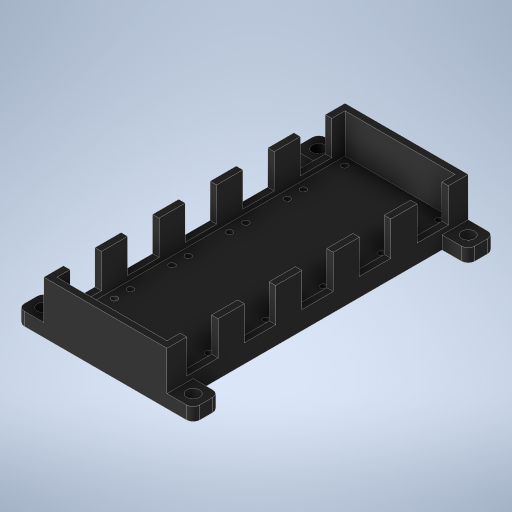
# Autodesk Inventor part: RelayCaseBottom
Saved by Autodesk Inventor 2024 (Build 280153000, 153)
## iProperties
Created: 2023-08-11
Part Number: RelayCaseBottom
Material: Rubber, Silicone
Document SubType Name: Modeling
Designer: 18179
Density: 1.25 g/cm^3
Appearance: Rubber - Black
Autodesk Inventor part; units mm, degrees
ref_plane "YZ Plane" through (0, 0, 0) normal (1, 0, 0) x (0, 1, 0)
ref_plane "XZ Plane" through (0, 0, 0) normal (0, 1, 0) x (-1, 0, 0)
ref_plane "XY Plane" through (0, 0, 0) normal (0, 0, 1) x (1, 0, 0)
sketch "0" plane through (0, 0, 0) normal (0, 0, 1) x (1, 0, 0)
  line L0 (-55.1011, 34.3581) -> (-55.1011, 26.7381)
  line L1 (-55.1011, 26.7381) -> (-57.6411, 26.7381)
  line L2 (-57.6411, 26.7381) -> (-57.6411, 34.3581)
  line L3 (-57.6411, 34.3581) -> (-55.1011, 34.3581)
  line L4 (-53.2169, 46.974) -> (-78.6169, 46.974)
  line L5 (-78.6169, 46.974) -> (-78.6169, -3.826)
  line L6 (-78.6169, -3.826) -> (-53.2169, -3.826)
  line L7 (-53.2169, -3.826) -> (-53.2169, 46.974)
  line L8 (-73.5115, 6.588) -> (-73.5115, 24.368)
  line L9 (-73.5115, 24.368) -> (-58.3223, 24.368)
  line L10 (-58.3223, 24.368) -> (-58.3223, 6.588)
  line L11 (-58.3223, 6.588) -> (-58.2969, 6.588)
  line L12 (-58.2969, 6.588) -> (-58.2969, -1.159)
  line L13 (-58.2969, -1.159) -> (-73.5369, -1.159)
  line L14 (-73.5369, -1.159) -> (-73.5369, 6.588)
  line L15 (-73.5369, 6.588) -> (-73.5115, 6.588)
  line L16 (-73.5369, 37.449) -> (-73.5369, 45.196)
  line L17 (-73.5369, 45.196) -> (-58.2969, 45.196)
  line L18 (-58.2969, 45.196) -> (-58.2969, 37.449)
  line L19 (-58.2969, 37.449) -> (-73.5369, 37.449)
  circle A0 centre (-75.9499, -1.2407) radius 1.524
  circle A1 centre (-55.8839, -1.2407) radius 1.524
  circle A2 centre (-75.9499, 44.3888) radius 1.524
  circle A3 centre (-55.8839, 44.3888) radius 1.524
  line L20 (-83.0411, 34.3581) -> (-83.0411, 26.7381)
  line L21 (-83.0411, 26.7381) -> (-85.5811, 26.7381)
  line L22 (-85.5811, 26.7381) -> (-85.5811, 34.3581)
  line L23 (-85.5811, 34.3581) -> (-83.0411, 34.3581)
  line L24 (-81.1569, 46.974) -> (-106.5569, 46.974)
  line L25 (-106.5569, 46.974) -> (-106.5569, -3.826)
  line L26 (-106.5569, -3.826) -> (-81.1569, -3.826)
  line L27 (-81.1569, -3.826) -> (-81.1569, 46.974)
  line L28 (-101.4515, 6.588) -> (-101.4515, 24.368)
  line L29 (-101.4515, 24.368) -> (-86.2623, 24.368)
  line L30 (-86.2623, 24.368) -> (-86.2623, 6.588)
  line L31 (-86.2623, 6.588) -> (-86.2369, 6.588)
  line L32 (-86.2369, 6.588) -> (-86.2369, -1.159)
  line L33 (-86.2369, -1.159) -> (-101.4769, -1.159)
  line L34 (-101.4769, -1.159) -> (-101.4769, 6.588)
  line L35 (-101.4769, 6.588) -> (-101.4515, 6.588)
  line L36 (-101.4769, 37.449) -> (-101.4769, 45.196)
  line L37 (-101.4769, 45.196) -> (-86.2369, 45.196)
  line L38 (-86.2369, 45.196) -> (-86.2369, 37.449)
  line L39 (-86.2369, 37.449) -> (-101.4769, 37.449)
  circle A4 centre (-103.8899, -1.2407) radius 1.524
  circle A5 centre (-83.8239, -1.2407) radius 1.524
  circle A6 centre (-103.8899, 44.3888) radius 1.524
  circle A7 centre (-83.8239, 44.3888) radius 1.524
  line L40 (-110.9811, 34.3581) -> (-110.9811, 26.7381)
  line L41 (-110.9811, 26.7381) -> (-113.5211, 26.7381)
  line L42 (-113.5211, 26.7381) -> (-113.5211, 34.3581)
  line L43 (-113.5211, 34.3581) -> (-110.9811, 34.3581)
  line L44 (-109.0969, 46.974) -> (-134.4969, 46.974)
  line L45 (-134.4969, 46.974) -> (-134.4969, -3.826)
  line L46 (-134.4969, -3.826) -> (-109.0969, -3.826)
  line L47 (-109.0969, -3.826) -> (-109.0969, 46.974)
  line L48 (-129.3915, 6.588) -> (-129.3915, 24.368)
  line L49 (-129.3915, 24.368) -> (-114.2023, 24.368)
  line L50 (-114.2023, 24.368) -> (-114.2023, 6.588)
  line L51 (-114.2023, 6.588) -> (-114.1769, 6.588)
  line L52 (-114.1769, 6.588) -> (-114.1769, -1.159)
  line L53 (-114.1769, -1.159) -> (-129.4169, -1.159)
  line L54 (-129.4169, -1.159) -> (-129.4169, 6.588)
  line L55 (-129.4169, 6.588) -> (-129.3915, 6.588)
  line L56 (-129.4169, 37.449) -> (-129.4169, 45.196)
  line L57 (-129.4169, 45.196) -> (-114.1769, 45.196)
  line L58 (-114.1769, 45.196) -> (-114.1769, 37.449)
  line L59 (-114.1769, 37.449) -> (-129.4169, 37.449)
  circle A8 centre (-131.8299, -1.2407) radius 1.524
  circle A9 centre (-111.7639, -1.2407) radius 1.524
  circle A10 centre (-131.8299, 44.3888) radius 1.524
  circle A11 centre (-111.7639, 44.3888) radius 1.524
  line L60 (-138.9211, 34.3581) -> (-138.9211, 26.7381)
  line L61 (-138.9211, 26.7381) -> (-141.4611, 26.7381)
  line L62 (-141.4611, 26.7381) -> (-141.4611, 34.3581)
  line L63 (-141.4611, 34.3581) -> (-138.9211, 34.3581)
  line L64 (-137.0369, 46.974) -> (-162.4369, 46.974)
  line L65 (-162.4369, 46.974) -> (-162.4369, -3.826)
  line L66 (-162.4369, -3.826) -> (-137.0369, -3.826)
  line L67 (-137.0369, -3.826) -> (-137.0369, 46.974)
  line L68 (-157.3315, 6.588) -> (-157.3315, 24.368)
  line L69 (-157.3315, 24.368) -> (-142.1423, 24.368)
  line L70 (-142.1423, 24.368) -> (-142.1423, 6.588)
  line L71 (-142.1423, 6.588) -> (-142.1169, 6.588)
  line L72 (-142.1169, 6.588) -> (-142.1169, -1.159)
  line L73 (-142.1169, -1.159) -> (-157.3569, -1.159)
  line L74 (-157.3569, -1.159) -> (-157.3569, 6.588)
  line L75 (-157.3569, 6.588) -> (-157.3315, 6.588)
  line L76 (-157.3569, 37.449) -> (-157.3569, 45.196)
  line L77 (-157.3569, 45.196) -> (-142.1169, 45.196)
  line L78 (-142.1169, 45.196) -> (-142.1169, 37.449)
  line L79 (-142.1169, 37.449) -> (-157.3569, 37.449)
  circle A12 centre (-159.7699, -1.2407) radius 1.524
  circle A13 centre (-139.7039, -1.2407) radius 1.524
  circle A14 centre (-159.7699, 44.3888) radius 1.524
  circle A15 centre (-139.7039, 44.3888) radius 1.524
  line L80 (-166.8611, 34.3581) -> (-166.8611, 26.7381)
  line L81 (-166.8611, 26.7381) -> (-169.4011, 26.7381)
  line L82 (-169.4011, 26.7381) -> (-169.4011, 34.3581)
  line L83 (-169.4011, 34.3581) -> (-166.8611, 34.3581)
  line L84 (-164.9769, 46.974) -> (-190.3769, 46.974)
  line L85 (-190.3769, 46.974) -> (-190.3769, -3.826)
  line L86 (-190.3769, -3.826) -> (-164.9769, -3.826)
  line L87 (-164.9769, -3.826) -> (-164.9769, 46.974)
  line L88 (-185.2715, 6.588) -> (-185.2715, 24.368)
  line L89 (-185.2715, 24.368) -> (-170.0823, 24.368)
  line L90 (-170.0823, 24.368) -> (-170.0823, 6.588)
  line L91 (-170.0823, 6.588) -> (-170.0569, 6.588)
  line L92 (-170.0569, 6.588) -> (-170.0569, -1.159)
  line L93 (-170.0569, -1.159) -> (-185.2969, -1.159)
  line L94 (-185.2969, -1.159) -> (-185.2969, 6.588)
  line L95 (-185.2969, 6.588) -> (-185.2715, 6.588)
  line L96 (-185.2969, 37.449) -> (-185.2969, 45.196)
  line L97 (-185.2969, 45.196) -> (-170.0569, 45.196)
  line L98 (-170.0569, 45.196) -> (-170.0569, 37.449)
  line L99 (-170.0569, 37.449) -> (-185.2969, 37.449)
  circle A16 centre (-187.7099, -1.2407) radius 1.524
  circle A17 centre (-167.6439, -1.2407) radius 1.524
  circle A18 centre (-187.7099, 44.3888) radius 1.524
  circle A19 centre (-167.6439, 44.3888) radius 1.524
  line L100 (-53.2169, -3.826) -> (-190.3769, -3.826)
  line L101 (-190.3769, -3.826) -> (-190.3769, 46.974)
  line L102 (-190.3769, 46.974) -> (-53.2169, 46.974)
  line L103 (-53.2169, 46.974) -> (-53.2169, -3.826)
  line L104 (-190.3769, 47.736) -> (-52.4549, 47.736)
  line L105 (-52.4549, 47.736) -> (-52.4549, -3.826)
  line L106 (-53.2169, -4.588) -> (-191.1389, -4.588)
  line L107 (-191.1389, -4.588) -> (-191.1389, 46.974)
  line L108 (-191.1389, -4.588) -> (-52.4549, -4.588)
  line L109 (-52.4549, -4.588) -> (-52.4549, 47.736)
  line L110 (-52.4549, 47.736) -> (-191.1389, 47.736)
  line L111 (-191.1389, 47.736) -> (-191.1389, -4.588)
  point P0 (-73.5369, 45.196)
  point P1 (-53.2169, -4.588)
  point P2 (-52.4549, -3.826)
  point P3 (-101.4769, 37.449)
  point P4 (-101.4769, -1.159)
  point P5 (-101.4769, 6.588)
  point P6 (-101.4515, 6.588)
  point P7 (-157.3569, 6.588)
  point P8 (-142.1169, 6.588)
  point P9 (-73.5115, 6.588)
  point P10 (-58.2969, -1.159)
  dimension "d0" = 25.4
  dimension "d1" = 50.8
  dimension "d2" = 3.048
  dimension "d3" = 1.8843
  dimension "d4" = 4.4243
  dimension "d5" = 5.08
  dimension "d6" = 5.08
  dimension "d7" = 5.1054
  dimension "d8" = 20.2946
  dimension "d9" = 20.32
  dimension "d10" = 20.32
  dimension "d11" = 7.62
  dimension "d12" = 12.6159
  dimension "d13" = 10.8379
  dimension "d14" = 3.0909
  dimension "d15" = 9.9901
  dimension "d16" = 35.5171
  dimension "d17" = 27.7701
  dimension "d18" = 20.1501
  dimension "d19" = 12.6159
  dimension "d20" = 0
  dimension "d21" = 38.1841
  dimension "d22" = 0
  dimension "d23" = 0
  dimension "d24" = 1.8843
  dimension "d25" = 7.62
  dimension "d26" = 1.8843
  dimension "d27" = 2.667
  dimension "d28" = 10.0307
  dimension "d29" = 2.667
  dimension "d30" = 35.5988
  dimension "d31" = 0
  dimension "d32" = 4.4243
  dimension "d33" = 7.62
  dimension "d34" = 4.4243
  dimension "d35" = 10.8379
  dimension "d36" = 5.08
  dimension "d37" = 3.0909
  dimension "d38" = 5.08
  dimension "d39" = 5.08
  dimension "d40" = 27.7701
  dimension "d41" = 5.08
  dimension "d42" = 35.5171
  dimension "d43" = 9.9901
  dimension "d44" = 5.1054
  dimension "d45" = 5.1054
  dimension "d46" = 27.7701
  dimension "d47" = 9.9901
  dimension "d48" = 20.2946
  dimension "d49" = 27.7701
  dimension "d50" = 20.2946
  dimension "d51" = 10.8379
  dimension "d52" = 20.32
  dimension "d53" = 3.0909
  dimension "d54" = 20.32
  dimension "d55" = 20.32
  dimension "d56" = 27.7701
  dimension "d57" = 20.32
  dimension "d58" = 35.5171
  dimension "d59" = 22.733
  dimension "d60" = 10.0307
  dimension "d61" = 22.733
  dimension "d62" = 35.5988
  dimension "d63" = 25.4
  constraints: 224 end point, 44 parallel, 38 perpendicular, 20 centre point, 15 equal radius, 14 collinear, 2 horizontal, 2 other
  measures "d0" distance between parallel lines of L7 L5
  measures "d1" distance between parallel lines of L6 L4
  measures "d2" diameter of A3
  measures "d3" distance between parallel lines of L0 L7
  measures "d4" distance between parallel lines of L2 L7
  measures "d5" distance between parallel lines of L7 L18
  measures "d6" distance between parallel lines of L12 L7
  measures "d7" distance between parallel lines of L7 L10
  measures "d8" distance between parallel lines of L7 L8
  measures "d9" distance between parallel lines of L7 L16
  measures "d10" distance between parallel lines of L14 L7
  measures "d11" distance between parallel lines of L1 L3
  measures "d12" distance between parallel lines of L3 L4
  measures "d13" distance between parallel lines of L3 L17
  measures "d14" distance between parallel lines of L3 L19
  measures "d15" distance between parallel lines of L3 L9
  measures "d16" distance between parallel lines of L13 L3
  measures "d17" distance between parallel lines of L3 L15
  measures "d18" distance between parallel lines of L11 L1
  measures "d19" distance from line of L7.end L3
  measures "d20" distance from line of L4.start L7
  measures "d21" distance from line of L7.start L3
  measures "d22" distance from line of L6.end L7
  measures "d23" distance from line of L0.start L3
  measures "d24" distance from line of L3.end L7
  measures "d25" distance from line of L0.end L3
  measures "d26" distance from line of L1.start L7
  measures "d27" distance from line of A3.centre L7
  measures "d28" distance from line of A3.centre L3
  measures "d29" distance from line of A1.centre L7
  measures "d30" distance from line of A1.centre L3
  measures "d31" distance from line of L2.end L3
  measures "d32" distance from line of L3.start L7
  measures "d33" distance from line of L2.start L3
  measures "d34" distance from line of L1.end L7
  measures "d35" distance from line of L18.start L3
  measures "d36" distance from line of L17.end L7
  measures "d37" distance from line of L18.end L3
  measures "d38" distance from line of L19.start L7
  measures "d39" distance from line of L11.end L7
  measures "d40" distance from line of L12.start L3
  measures "d41" distance from line of L13.start L7
  measures "d42" distance from line of L12.end L3
  measures "d43" distance from line of L10.start L3
  measures "d44" distance from line of L9.end L7
  measures "d45" distance from line of L11.start L7
  measures "d46" distance from line of L10.end L3
  measures "d47" distance from line of L8.end L3
  measures "d48" distance from line of L9.start L7
  measures "d49" distance from line of L8.start L3
  measures "d50" distance from line of L15.end L7
  measures "d51" distance from line of L16.end L3
  measures "d52" distance from line of L17.start L7
  measures "d53" distance from line of L16.start L3
  measures "d54" distance from line of L19.end L7
  measures "d55" distance from line of L15.start L7
  measures "d56" distance from line of L14.end L3
  measures "d57" distance from line of L13.end L7
  measures "d58" distance from line of L14.start L3
  measures "d59" distance from line of A2.centre L7
  measures "d60" distance from line of A2.centre L3
  measures "d61" distance from line of A0.centre L7
  measures "d62" distance from line of A0.centre L3
  measures "d63" distance from line of L4.end L7
extrude "Extrusion1" add sketch "0" along normal blind 3.175 contours L0 L1 L2 L3 | L7 L6 L5 L4 | L5 L100 L27 L102 | L27 L26 L25 L24 | L25 L100 L47 L102 | L47 L46 L45 L44 | L45 L100 L67 L102 | L67 L66 L65 L64 | L65 L100 L87 L102 | L87 L86 L85 L84 | L20 L21 L22 L23 | L40 L41 L42 L43 | L60 L61 L62 L63 | L80 L81 L82 L83 | L104 L105 L109 L108 L106 L107 L111 L110
sketch "Sketch10" plane through (0, 0, 3.175) normal (0, 0, 1) x (1, 0, 0)
  line L0 (-191.1389, 47.736) -> (-191.1389, -4.588) projected
  line L1 (-191.1389, -4.588) -> (-52.4549, -4.588) projected
  line L2 (-52.4549, -4.588) -> (-52.4549, 47.736) projected
  line L3 (-52.4549, 47.736) -> (-191.1389, 47.736) projected
  line L4 (-101.4769, -1.159) -> (-101.4769, 6.588) projected
  line L5 (-101.4769, 6.588) -> (-101.4515, 6.588) projected
  line L6 (-101.4515, 6.588) -> (-101.4515, 24.368) projected
  line L7 (-101.4515, 24.368) -> (-86.2623, 24.368) projected
  line L8 (-86.2623, 24.368) -> (-86.2623, 6.588) projected
  line L9 (-86.2623, 6.588) -> (-86.2369, 6.588) projected
  line L10 (-86.2369, 6.588) -> (-86.2369, -1.159) projected
  line L11 (-86.2369, -1.159) -> (-101.4769, -1.159) projected
  line L12 (-86.2369, 37.449) -> (-101.4769, 37.449) projected
  line L13 (-101.4769, 37.449) -> (-101.4769, 45.196) projected
  line L14 (-101.4769, 45.196) -> (-86.2369, 45.196) projected
  line L15 (-86.2369, 45.196) -> (-86.2369, 37.449) projected
  circle A0 centre (-103.8899, 44.3888) radius 1.524 projected
  circle A1 centre (-83.8239, 44.3888) radius 1.524 projected
  circle A2 centre (-103.8899, -1.2407) radius 1.524 projected
  circle A3 centre (-83.8239, -1.2407) radius 1.524 projected
  line L16 (-157.3569, -1.159) -> (-157.3569, 6.588) projected
  line L17 (-157.3569, 6.588) -> (-157.3315, 6.588) projected
  line L18 (-157.3315, 6.588) -> (-157.3315, 24.368) projected
  line L19 (-157.3315, 24.368) -> (-142.1423, 24.368) projected
  line L20 (-142.1423, 24.368) -> (-142.1423, 6.588) projected
  line L21 (-142.1423, 6.588) -> (-142.1169, 6.588) projected
  line L22 (-142.1169, 6.588) -> (-142.1169, -1.159) projected
  line L23 (-142.1169, -1.159) -> (-157.3569, -1.159) projected
  line L24 (-142.1169, 37.449) -> (-157.3569, 37.449) projected
  line L25 (-157.3569, 37.449) -> (-157.3569, 45.196) projected
  line L26 (-157.3569, 45.196) -> (-142.1169, 45.196) projected
  line L27 (-142.1169, 45.196) -> (-142.1169, 37.449) projected
  circle A4 centre (-159.7699, 44.3888) radius 1.524 projected
  circle A5 centre (-139.7039, 44.3888) radius 1.524 projected
  circle A6 centre (-159.7699, -1.2407) radius 1.524 projected
  circle A7 centre (-139.7039, -1.2407) radius 1.524 projected
  line L28 (-185.2969, -1.159) -> (-185.2969, 6.588) projected
  line L29 (-185.2969, 6.588) -> (-185.2715, 6.588) projected
  line L30 (-185.2715, 6.588) -> (-185.2715, 24.368) projected
  line L31 (-185.2715, 24.368) -> (-170.0823, 24.368) projected
  line L32 (-170.0823, 24.368) -> (-170.0823, 6.588) projected
  line L33 (-170.0823, 6.588) -> (-170.0569, 6.588) projected
  line L34 (-170.0569, 6.588) -> (-170.0569, -1.159) projected
  line L35 (-170.0569, -1.159) -> (-185.2969, -1.159) projected
  line L36 (-170.0569, 37.449) -> (-185.2969, 37.449) projected
  line L37 (-185.2969, 37.449) -> (-185.2969, 45.196) projected
  line L38 (-185.2969, 45.196) -> (-170.0569, 45.196) projected
  line L39 (-170.0569, 45.196) -> (-170.0569, 37.449) projected
  circle A8 centre (-187.7099, 44.3888) radius 1.524 projected
  circle A9 centre (-167.6439, 44.3888) radius 1.524 projected
  circle A10 centre (-187.7099, -1.2407) radius 1.524 projected
  circle A11 centre (-167.6439, -1.2407) radius 1.524 projected
  circle A12 centre (-111.7639, -1.2407) radius 1.524 projected
  circle A13 centre (-131.8299, -1.2407) radius 1.524 projected
  circle A14 centre (-111.7639, 44.3888) radius 1.524 projected
  circle A15 centre (-131.8299, 44.3888) radius 1.524 projected
  line L40 (-114.1769, 37.449) -> (-129.4169, 37.449) projected
  line L41 (-129.4169, 37.449) -> (-129.4169, 45.196) projected
  line L42 (-129.4169, 45.196) -> (-114.1769, 45.196) projected
  line L43 (-114.1769, 45.196) -> (-114.1769, 37.449) projected
  line L44 (-129.4169, -1.159) -> (-129.4169, 6.588) projected
  line L45 (-129.4169, 6.588) -> (-129.3915, 6.588) projected
  line L46 (-129.3915, 6.588) -> (-129.3915, 24.368) projected
  line L47 (-129.3915, 24.368) -> (-114.2023, 24.368) projected
  line L48 (-114.2023, 24.368) -> (-114.2023, 6.588) projected
  line L49 (-114.2023, 6.588) -> (-114.1769, 6.588) projected
  line L50 (-114.1769, 6.588) -> (-114.1769, -1.159) projected
  line L51 (-114.1769, -1.159) -> (-129.4169, -1.159) projected
  line L52 (-73.5115, 6.588) -> (-73.5115, 24.368) projected
  line L53 (-73.5115, 24.368) -> (-58.3223, 24.368) projected
  line L54 (-58.3223, 24.368) -> (-58.3223, 6.588) projected
  line L55 (-58.3223, 6.588) -> (-58.2969, 6.588) projected
  line L56 (-58.2969, 6.588) -> (-58.2969, -1.159) projected
  line L57 (-58.2969, -1.159) -> (-73.5369, -1.159) projected
  line L58 (-73.5369, -1.159) -> (-73.5369, 6.588) projected
  line L59 (-73.5369, 6.588) -> (-73.5115, 6.588) projected
  line L60 (-73.5369, 37.449) -> (-73.5369, 45.196) projected
  line L61 (-73.5369, 45.196) -> (-58.2969, 45.196) projected
  line L62 (-58.2969, 45.196) -> (-58.2969, 37.449) projected
  line L63 (-58.2969, 37.449) -> (-73.5369, 37.449) projected
  circle A16 centre (-55.8839, 44.3888) radius 1.524 projected
  circle A17 centre (-75.9499, 44.3888) radius 1.524 projected
  circle A18 centre (-55.8839, -1.2407) radius 1.524 projected
  circle A19 centre (-75.9499, -1.2407) radius 1.524 projected
  line L64 (-191.6865, 48.2837) -> (-191.6865, -5.1356)
  line L65 (-191.6865, -5.1356) -> (-51.9072, -5.1356)
  line L66 (-51.9072, -5.1356) -> (-51.9072, 48.2837)
  line L67 (-51.9072, 48.2837) -> (-191.6865, 48.2837)
  line L68 (-194.8615, 51.4587) -> (-194.8615, -8.3106)
  line L69 (-194.8615, -8.3106) -> (-48.7322, -8.3106)
  line L70 (-48.7322, -8.3106) -> (-48.7322, 51.4587)
  line L71 (-48.7322, 51.4587) -> (-194.8615, 51.4587)
  line L72 (-185.2969, 45.196) -> (-170.0569, 45.196)
  line L73 (-170.0569, 45.196) -> (-170.0569, 51.4587)
  line L74 (-170.0569, 51.4587) -> (-185.2969, 51.4587)
  line L75 (-185.2969, 51.4587) -> (-185.2969, 45.196)
  line L76 (-157.3569, 45.196) -> (-142.1169, 45.196)
  line L77 (-142.1169, 45.196) -> (-142.1169, 51.4587)
  line L78 (-142.1169, 51.4587) -> (-157.3569, 51.4587)
  line L79 (-157.3569, 51.4587) -> (-157.3569, 45.196)
  line L80 (-114.1769, 37.449) -> (-129.4169, 37.449)
  line L81 (-129.4169, 37.449) -> (-129.4169, 51.4587)
  line L82 (-129.4169, 51.4587) -> (-114.1769, 51.4587)
  line L83 (-114.1769, 51.4587) -> (-114.1769, 37.449)
  line L84 (-86.2369, 37.449) -> (-101.4769, 37.449)
  line L85 (-101.4769, 37.449) -> (-101.4769, 51.4587)
  line L86 (-101.4769, 51.4587) -> (-86.2369, 51.4587)
  line L87 (-86.2369, 51.4587) -> (-86.2369, 37.449)
  line L88 (-73.5369, 37.449) -> (-58.2969, 37.449)
  line L89 (-58.2969, 37.449) -> (-58.2969, 51.4587)
  line L90 (-58.2969, 51.4587) -> (-73.5369, 51.4587)
  line L91 (-73.5369, 51.4587) -> (-73.5369, 37.449)
  line L92 (-58.2969, -1.159) -> (-73.5369, -1.159)
  line L93 (-73.5369, -1.159) -> (-73.5369, -8.3106)
  line L94 (-73.5369, -8.3106) -> (-58.2969, -8.3106)
  line L95 (-58.2969, -8.3106) -> (-58.2969, -1.159)
  line L96 (-86.2369, -1.159) -> (-101.4769, -1.159)
  line L97 (-101.4769, -1.159) -> (-101.4769, -8.3106)
  line L98 (-101.4769, -8.3106) -> (-86.2369, -8.3106)
  line L99 (-86.2369, -8.3106) -> (-86.2369, -1.159)
  line L100 (-114.1769, -1.159) -> (-129.4169, -1.159)
  line L101 (-129.4169, -1.159) -> (-129.4169, -5.1356)
  line L102 (-129.4169, -5.1356) -> (-114.1769, -5.1356)
  line L103 (-114.1769, -5.1356) -> (-114.1769, -1.159)
  line L104 (-129.4169, -3.1473) -> (-114.1769, -3.1473)
  line L105 (-114.1769, -3.1473) -> (-114.1769, -8.3106)
  line L106 (-114.1769, -8.3106) -> (-129.4169, -8.3106)
  line L107 (-129.4169, -8.3106) -> (-129.4169, -3.1473)
  line L108 (-142.1169, -1.159) -> (-157.3569, -1.159)
  line L109 (-157.3569, -1.159) -> (-157.3569, -5.1356)
  line L110 (-157.3569, -5.1356) -> (-142.1169, -5.1356)
  line L111 (-142.1169, -5.1356) -> (-142.1169, -1.159)
  line L112 (-170.0569, -1.159) -> (-185.2969, -1.159)
  line L113 (-185.2969, -1.159) -> (-185.2969, -8.3106)
  line L114 (-185.2969, -8.3106) -> (-170.0569, -8.3106)
  line L115 (-170.0569, -8.3106) -> (-170.0569, -1.159)
  line L116 (-157.3569, -3.1473) -> (-142.1169, -3.1473)
  line L117 (-142.1169, -3.1473) -> (-142.1169, -8.3106)
  line L118 (-142.1169, -8.3106) -> (-157.3569, -8.3106)
  line L119 (-157.3569, -8.3106) -> (-157.3569, -3.1473)
  point P0 (0, 0)
  point P1 (-185.2969, 48.2837)
  point P2 (-185.2969, -5.1356)
  point P3 (-170.0569, -5.1356)
  point P4 (-101.4769, -5.1356)
  point P5 (-86.2369, -5.1356)
  point P6 (-73.5369, -5.1356)
  point P7 (-58.2969, -5.1356)
  point P8 (-58.2969, 48.2837)
  point P9 (-73.5369, 48.2837)
  point P10 (-86.2369, 48.2837)
  point P11 (-101.4769, 48.2837)
  point P12 (-114.1769, 48.2837)
  point P13 (-129.4169, 48.2837)
  point P14 (-142.1169, 48.2837)
  point P15 (-157.3569, 48.2837)
  point P16 (-170.0569, 48.2837)
  dimension "d367" = 3.175
  constraints: 112 end point, 24 parallel, 18 point on line, 12 horizontal, 12 perpendicular, 2 midpoint, 6 other
  measures "d367" distance between parallel lines of L67 L71
extrude "Extrusion7" add sketch "Sketch10" along normal blind 19.05 contours L67 L64 L65 L113 L69 L68 L71 L75 | L73 L71 L79 L67 | L65 L119 L69 L115 | L77 L71 L81 L67 | L65 L107 L69 L117 | L83 L71 L85 L67 | L65 L97 L69 L105 | L87 L71 L91 L67 | L65 L93 L69 L99 | L89 L71 L70 L69 L95 L65 L66 L67
sketch "Sketch11" plane through (0, 0, 3.175) normal (0, 0, 1) x (1, 0, 0)
  line L0 (-191.6865, 48.2837) -> (-185.2969, 48.2837) projected
  line L1 (-185.2969, 48.2837) -> (-185.2969, 51.4587) projected
  line L2 (-185.2969, 51.4587) -> (-194.8615, 51.4587) projected
  line L3 (-194.8615, 51.4587) -> (-194.8615, -8.3106) projected
  line L4 (-194.8615, -8.3106) -> (-185.2969, -8.3106) projected
  line L5 (-185.2969, -8.3106) -> (-185.2969, -5.1356) projected
  line L6 (-185.2969, -5.1356) -> (-191.6865, -5.1356) projected
  line L7 (-191.6865, -5.1356) -> (-191.6865, 48.2837) projected
  line L8 (-157.3569, 51.4587) -> (-170.0569, 51.4587) projected
  line L9 (-170.0569, 51.4587) -> (-170.0569, 48.2837) projected
  line L10 (-170.0569, 48.2837) -> (-157.3569, 48.2837) projected
  line L11 (-157.3569, 48.2837) -> (-157.3569, 51.4587) projected
  line L12 (-129.4169, 51.4587) -> (-142.1169, 51.4587) projected
  line L13 (-142.1169, 51.4587) -> (-142.1169, 48.2837) projected
  line L14 (-142.1169, 48.2837) -> (-129.4169, 48.2837) projected
  line L15 (-129.4169, 48.2837) -> (-129.4169, 51.4587) projected
  line L16 (-101.4769, 51.4587) -> (-114.1769, 51.4587) projected
  line L17 (-114.1769, 51.4587) -> (-114.1769, 48.2837) projected
  line L18 (-114.1769, 48.2837) -> (-101.4769, 48.2837) projected
  line L19 (-101.4769, 48.2837) -> (-101.4769, 51.4587) projected
  line L20 (-73.5369, 51.4587) -> (-86.2369, 51.4587) projected
  line L21 (-73.5369, 51.4587) -> (-86.2369, 51.4587) projected
  line L22 (-86.2369, 51.4587) -> (-86.2369, 48.2837) projected
  line L23 (-86.2369, 48.2837) -> (-73.5369, 48.2837) projected
  line L24 (-73.5369, 48.2837) -> (-73.5369, 51.4587) projected
  line L25 (-51.9072, -5.1356) -> (-58.2969, -5.1356) projected
  line L26 (-58.2969, -5.1356) -> (-58.2969, -8.3106) projected
  line L27 (-58.2969, -8.3106) -> (-48.7322, -8.3106) projected
  line L28 (-48.7322, -8.3106) -> (-48.7322, 51.4587) projected
  line L29 (-48.7322, 51.4587) -> (-58.2969, 51.4587) projected
  line L30 (-58.2969, 51.4587) -> (-58.2969, 48.2837) projected
  line L31 (-58.2969, 48.2837) -> (-51.9072, 48.2837) projected
  line L32 (-51.9072, 48.2837) -> (-51.9072, -5.1356) projected
  line L33 (-86.2369, -8.3106) -> (-73.5369, -8.3106) projected
  line L34 (-73.5369, -8.3106) -> (-73.5369, -5.1356) projected
  line L35 (-73.5369, -5.1356) -> (-86.2369, -5.1356) projected
  line L36 (-86.2369, -5.1356) -> (-86.2369, -8.3106) projected
  line L37 (-114.1769, -8.3106) -> (-101.4769, -8.3106) projected
  line L38 (-101.4769, -8.3106) -> (-101.4769, -5.1356) projected
  line L39 (-101.4769, -5.1356) -> (-114.1769, -5.1356) projected
  line L40 (-114.1769, -5.1356) -> (-114.1769, -8.3106) projected
  line L41 (-129.4169, -5.1356) -> (-142.1169, -5.1356) projected
  line L42 (-142.1169, -8.3106) -> (-129.4169, -8.3106) projected
  line L43 (-129.4169, -8.3106) -> (-129.4169, -5.1356) projected
  line L44 (-129.4169, -5.1356) -> (-142.1169, -5.1356) projected
  line L45 (-142.1169, -5.1356) -> (-142.1169, -8.3106) projected
  line L46 (-157.3569, -5.1356) -> (-170.0569, -5.1356) projected
  line L47 (-170.0569, -5.1356) -> (-170.0569, -8.3106) projected
  line L48 (-170.0569, -8.3106) -> (-157.3569, -8.3106) projected
  line L49 (-157.3569, -8.3106) -> (-157.3569, -5.1356) projected
  line L50 (-185.2969, 48.2837) -> (-170.0569, 48.2837)
  line L51 (-170.0569, 48.2837) -> (-170.0569, 51.4587)
  line L52 (-170.0569, 51.4587) -> (-185.2969, 51.4587)
  line L53 (-185.2969, 51.4587) -> (-185.2969, 48.2837)
  line L54 (-157.3569, 48.2837) -> (-142.1169, 48.2837)
  line L55 (-142.1169, 48.2837) -> (-142.1169, 51.4587)
  line L56 (-142.1169, 51.4587) -> (-157.3569, 51.4587)
  line L57 (-157.3569, 51.4587) -> (-157.3569, 48.2837)
  line L58 (-129.4169, 48.2837) -> (-114.1769, 48.2837)
  line L59 (-114.1769, 48.2837) -> (-114.1769, 51.4587)
  line L60 (-114.1769, 51.4587) -> (-129.4169, 51.4587)
  line L61 (-129.4169, 51.4587) -> (-129.4169, 48.2837)
  line L62 (-121.7969, 51.4587) -> (-121.7969, 18.9884)
  line L63 (-194.8615, 21.574) -> (-174.664, 21.574)
  line L64 (-58.2969, 48.2837) -> (-73.5369, 48.2837)
  line L65 (-73.5369, 51.4587) -> (-58.2969, 51.4587)
  line L66 (-86.2369, 48.2837) -> (-101.4769, 48.2837)
  line L67 (-101.4769, 51.4587) -> (-86.2369, 51.4587)
  line L68 (-114.1769, 48.2837) -> (-129.4169, 48.2837)
  line L69 (-129.4169, 51.4587) -> (-114.1769, 51.4587)
  line L70 (-185.2969, -5.1356) -> (-170.0569, -5.1356)
  line L71 (-170.0569, -8.3106) -> (-185.2969, -8.3106)
  line L72 (-157.3569, -5.1356) -> (-142.1169, -5.1356)
  line L73 (-142.1169, -8.3106) -> (-157.3569, -8.3106)
  line L74 (-129.4169, -5.1356) -> (-114.1769, -5.1356)
  line L75 (-114.1769, -8.3106) -> (-129.4169, -8.3106)
  line L76 (-73.5369, -8.3106) -> (-58.2969, -8.3106)
  line L77 (-58.2969, -5.1356) -> (-73.5369, -5.1356)
  line L78 (-101.4769, -8.3106) -> (-86.2369, -8.3106)
  line L79 (-86.2369, -5.1356) -> (-101.4769, -5.1356)
  point P0 (0, 0)
  constraints: 60 end point, 21 symmetric about line, 6 parallel, 4 horizontal, 3 perpendicular, 2 midpoint, 1 vertical
extrude "Extrusion8" add sketch "Sketch11" along normal blind 2.54 contours L1 L52 L9 L50 | L11 L56 L13 L54 | L70 L47 L71 L5 | L15 L60 L62 L58 | L72 L45 L73 L49 | L62 L60 L17 L58 | L74 L40 L75 L43 | L19 L67 L22 L66 | L79 L36 L78 L38 | L24 L65 L30 L64 | L77 L26 L76 L34
sketch "Sketch12" plane through (0, 0, 0) normal (0, 0, -1) x (-1, 0, 0)
  line L0 (194.8615, -8.3106) -> (48.7322, -8.3106) projected
  line L1 (194.8615, 51.4587) -> (194.8615, -8.3106) projected
  line L2 (191.1389, 47.736) -> (191.1389, -4.588) projected
  line L3 (191.1389, -4.588) -> (52.4549, -4.588) projected
  line L4 (52.4549, -4.588) -> (52.4549, 47.736) projected
  line L5 (52.4549, 47.736) -> (191.1389, 47.736) projected
  line L6 (191.1389, 47.736) -> (191.1389, -4.588) projected
  line L7 (52.4549, 47.736) -> (191.1389, 47.736) projected
  line L8 (52.4549, -4.588) -> (52.4549, 47.736) projected
  line L9 (191.1389, -4.588) -> (52.4549, -4.588) projected
  line L10 (101.4769, -1.159) -> (101.4769, 6.588) projected
  line L11 (86.2369, -1.159) -> (101.4769, -1.159) projected
  line L12 (86.2369, 6.588) -> (86.2369, -1.159) projected
  line L13 (86.2623, 6.588) -> (86.2369, 6.588) projected
  line L14 (86.2623, 24.368) -> (86.2623, 6.588) projected
  line L15 (101.4515, 24.368) -> (86.2623, 24.368) projected
  line L16 (101.4515, 6.588) -> (101.4515, 24.368) projected
  line L17 (101.4769, 6.588) -> (101.4515, 6.588) projected
  line L18 (86.2369, 37.449) -> (101.4769, 37.449) projected
  line L19 (86.2369, 45.196) -> (86.2369, 37.449) projected
  line L20 (101.4769, 45.196) -> (86.2369, 45.196) projected
  line L21 (101.4769, 37.449) -> (101.4769, 45.196) projected
  circle A0 centre (103.8899, 44.3888) radius 1.524 projected
  circle A1 centre (83.8239, 44.3888) radius 1.524 projected
  circle A2 centre (103.8899, -1.2407) radius 1.524 projected
  circle A3 centre (83.8239, -1.2407) radius 1.524 projected
  line L22 (157.3569, -1.159) -> (157.3569, 6.588) projected
  line L23 (142.1169, -1.159) -> (157.3569, -1.159) projected
  line L24 (142.1169, 6.588) -> (142.1169, -1.159) projected
  line L25 (142.1423, 6.588) -> (142.1169, 6.588) projected
  line L26 (142.1423, 24.368) -> (142.1423, 6.588) projected
  line L27 (157.3315, 24.368) -> (142.1423, 24.368) projected
  line L28 (157.3315, 6.588) -> (157.3315, 24.368) projected
  line L29 (157.3569, 6.588) -> (157.3315, 6.588) projected
  line L30 (142.1169, 37.449) -> (157.3569, 37.449) projected
  line L31 (142.1169, 45.196) -> (142.1169, 37.449) projected
  line L32 (157.3569, 45.196) -> (142.1169, 45.196) projected
  line L33 (157.3569, 37.449) -> (157.3569, 45.196) projected
  circle A4 centre (159.7699, 44.3888) radius 1.524 projected
  circle A5 centre (139.7039, 44.3888) radius 1.524 projected
  circle A6 centre (159.7699, -1.2407) radius 1.524 projected
  circle A7 centre (139.7039, -1.2407) radius 1.524 projected
  line L34 (185.2969, -1.159) -> (185.2969, 6.588) projected
  line L35 (170.0569, -1.159) -> (185.2969, -1.159) projected
  line L36 (170.0569, 6.588) -> (170.0569, -1.159) projected
  line L37 (170.0823, 6.588) -> (170.0569, 6.588) projected
  line L38 (170.0823, 24.368) -> (170.0823, 6.588) projected
  line L39 (185.2715, 24.368) -> (170.0823, 24.368) projected
  line L40 (185.2715, 6.588) -> (185.2715, 24.368) projected
  line L41 (185.2969, 6.588) -> (185.2715, 6.588) projected
  line L42 (170.0569, 37.449) -> (185.2969, 37.449) projected
  line L43 (170.0569, 45.196) -> (170.0569, 37.449) projected
  line L44 (185.2969, 45.196) -> (170.0569, 45.196) projected
  line L45 (185.2969, 37.449) -> (185.2969, 45.196) projected
  circle A8 centre (187.7099, 44.3888) radius 1.524 projected
  circle A9 centre (167.6439, 44.3888) radius 1.524 projected
  circle A10 centre (187.7099, -1.2407) radius 1.524 projected
  circle A11 centre (167.6439, -1.2407) radius 1.524 projected
  circle A12 centre (111.7639, -1.2407) radius 1.524 projected
  circle A13 centre (131.8299, -1.2407) radius 1.524 projected
  circle A14 centre (111.7639, 44.3888) radius 1.524 projected
  circle A15 centre (131.8299, 44.3888) radius 1.524 projected
  line L46 (114.1769, 37.449) -> (129.4169, 37.449) projected
  line L47 (114.1769, 45.196) -> (114.1769, 37.449) projected
  line L48 (129.4169, 45.196) -> (114.1769, 45.196) projected
  line L49 (129.4169, 37.449) -> (129.4169, 45.196) projected
  line L50 (129.4169, -1.159) -> (129.4169, 6.588) projected
  line L51 (114.1769, -1.159) -> (129.4169, -1.159) projected
  line L52 (114.1769, 6.588) -> (114.1769, -1.159) projected
  line L53 (114.2023, 6.588) -> (114.1769, 6.588) projected
  line L54 (114.2023, 24.368) -> (114.2023, 6.588) projected
  line L55 (129.3915, 24.368) -> (114.2023, 24.368) projected
  line L56 (129.3915, 6.588) -> (129.3915, 24.368) projected
  line L57 (129.4169, 6.588) -> (129.3915, 6.588) projected
  line L58 (73.5115, 6.588) -> (73.5115, 24.368) projected
  line L59 (73.5369, 6.588) -> (73.5115, 6.588) projected
  line L60 (73.5369, -1.159) -> (73.5369, 6.588) projected
  line L61 (58.2969, -1.159) -> (73.5369, -1.159) projected
  line L62 (58.2969, 6.588) -> (58.2969, -1.159) projected
  line L63 (58.3223, 6.588) -> (58.2969, 6.588) projected
  line L64 (58.3223, 24.368) -> (58.3223, 6.588) projected
  line L65 (73.5115, 24.368) -> (58.3223, 24.368) projected
  line L66 (73.5369, 37.449) -> (73.5369, 45.196) projected
  line L67 (58.2969, 37.449) -> (73.5369, 37.449) projected
  line L68 (58.2969, 45.196) -> (58.2969, 37.449) projected
  line L69 (73.5369, 45.196) -> (58.2969, 45.196) projected
  circle A16 centre (55.8839, 44.3888) radius 1.524 projected
  circle A17 centre (75.9499, 44.3888) radius 1.524 projected
  circle A18 centre (55.8839, -1.2407) radius 1.524 projected
  circle A19 centre (75.9499, -1.2407) radius 1.524 projected
  line L70 (48.7322, 51.4587) -> (194.8615, 51.4587) projected
  line L71 (48.7322, -8.3106) -> (48.7322, 51.4587) projected
  line L72 (121.7969, -8.3106) -> (121.7969, -13.957)
  line L73 (48.7322, -8.3106) -> (61.4322, -8.3106)
  line L74 (61.4322, -8.3106) -> (61.4322, -17.8356)
  line L75 (58.2572, -21.0106) -> (51.9072, -21.0106)
  line L76 (48.7322, -17.8356) -> (48.7322, -8.3106)
  line L77 (48.7322, 51.4587) -> (61.4322, 51.4587)
  line L78 (61.4322, 51.4587) -> (61.4322, 60.9837)
  line L79 (58.2572, 64.1587) -> (51.9072, 64.1587)
  line L80 (48.7322, 60.9837) -> (48.7322, 51.4587)
  circle A20 centre (55.0822, 57.8087) radius 3.175
  circle A21 centre (55.0822, -14.6606) radius 3.175
  arc A22 (58.2572, -21.0106) -> (61.4322, -17.8356) centre (58.2572, -17.8356) ccw
  arc A23 (48.7322, -17.8356) -> (51.9072, -21.0106) centre (51.9072, -17.8356) ccw
  arc A24 (51.9072, 64.1587) -> (48.7322, 60.9837) centre (51.9072, 60.9837) ccw
  arc A25 (61.4322, 60.9837) -> (58.2572, 64.1587) centre (58.2572, 60.9837) ccw
  line L81 (182.1615, -8.3106) -> (182.1615, -17.8356)
  line L82 (185.3365, -21.0106) -> (191.6865, -21.0106)
  line L83 (194.8615, -17.8356) -> (194.8615, -8.3106)
  line L84 (182.1615, 51.4587) -> (182.1615, 60.9837)
  line L85 (185.3365, 64.1587) -> (191.6865, 64.1587)
  line L86 (194.8615, 60.9837) -> (194.8615, 51.4587)
  circle A26 centre (188.5115, 57.8087) radius 3.175
  circle A27 centre (188.5115, -14.6606) radius 3.175
  arc A28 (182.1615, -17.8356) -> (185.3365, -21.0106) centre (185.3365, -17.8356) ccw
  arc A29 (191.6865, -21.0106) -> (194.8615, -17.8356) centre (191.6865, -17.8356) ccw
  arc A30 (194.8615, 60.9837) -> (191.6865, 64.1587) centre (191.6865, 60.9837) ccw
  arc A31 (185.3365, 64.1587) -> (182.1615, 60.9837) centre (185.3365, 60.9837) ccw
  point P0 (0, 0)
  point P1 (61.4322, -21.0106)
  point P2 (48.7322, -21.0106)
  point P3 (61.4322, 64.1587)
  point P4 (48.7322, 64.1587)
  dimension "d372" = 12.7
  dimension "d373" = 12.7
  dimension "d374" = 12.7
  dimension "d375" = 12.7
  dimension "d376" = 6.35
  dimension "d377" = 6.35
  dimension "d378" = 3.175
  constraints: 30 end point, 16 point on circle, 16 symmetric about line, 12 centre point, 8 point on line, 8 tangent, 4 parallel, 3 equal radius, 2 horizontal, 2 perpendicular, 1 midpoint, 1 vertical, 6 other
  measures "d372" distance of point (61.432, -21.011) point (48.732, -21.011)
  measures "d373" distance of L73.end point (61.432, -21.011)
  measures "d374" distance of point (48.732, 64.159) point (61.432, 64.159)
  measures "d375" distance of point (61.432, 64.159) L77.end
  measures "d376" diameter of A20
  measures "d377" diameter of A21
  measures "d378" radius of A22
extrude "Extrusion9" add sketch "Sketch12" against normal blind 3.175 contours L83 A29 L82 A28 L81 L0 | L0 L71 L70 L1 | L70 L84 A31 L85 A30 L86 | L74 A22 L75 A23 L76 L0 | L70 L80 A24 L79 A25 L78 | L11 L12 L13 L14 L15 L16 L17 L10 | L19 L20 L21 L18 | L23 L24 L25 L26 L27 L28 L29 L22 | L31 L32 L33 L30 | L35 L36 L37 L38 L39 L40 L41 L34 | L43 L44 L45 L42 | L47 L48 L49 L46 | L51 L52 L53 L54 L55 L56 L57 L50 | L59 L60 L61 L62 L63 L64 L65 L58 | L67 L68 L69 L66
sketch "Sketch13" plane through (0, 0, 0) normal (0, 0, -1) x (-1, 0, 0)
  circle A0 centre (188.5115, 57.8087) radius 3.175 projected
  circle A1 centre (55.0822, 57.8087) radius 3.175 projected
  circle A2 centre (55.0822, -14.6606) radius 3.175 projected
  circle A3 centre (188.5115, -14.6606) radius 3.175 projected
  line L0 (194.8615, -17.8356) -> (194.8615, 60.9837) projected
  arc A4 (194.8615, 60.9837) -> (191.6865, 64.1587) centre (191.6865, 60.9837) ccw projected
  line L1 (191.6865, 64.1587) -> (185.3365, 64.1587) projected
  arc A5 (185.3365, 64.1587) -> (182.1615, 60.9837) centre (185.3365, 60.9837) ccw projected
  line L2 (182.1615, 60.9837) -> (182.1615, 51.4587) projected
  line L3 (182.1615, 51.4587) -> (61.4322, 51.4587) projected
  line L4 (61.4322, 51.4587) -> (61.4322, 60.9837) projected
  arc A6 (61.4322, 60.9837) -> (58.2572, 64.1587) centre (58.2572, 60.9837) ccw projected
  line L5 (58.2572, 64.1587) -> (51.9072, 64.1587) projected
  arc A7 (51.9072, 64.1587) -> (48.7322, 60.9837) centre (51.9072, 60.9837) ccw projected
  line L6 (48.7322, 60.9837) -> (48.7322, -17.8356) projected
  arc A8 (48.7322, -17.8356) -> (51.9072, -21.0106) centre (51.9072, -17.8356) ccw projected
  line L7 (51.9072, -21.0106) -> (58.2572, -21.0106) projected
  arc A9 (58.2572, -21.0106) -> (61.4322, -17.8356) centre (58.2572, -17.8356) ccw projected
  line L8 (61.4322, -17.8356) -> (61.4322, -8.3106) projected
  line L9 (61.4322, -8.3106) -> (182.1615, -8.3106) projected
  line L10 (182.1615, -8.3106) -> (182.1615, -17.8356) projected
  arc A10 (182.1615, -17.8356) -> (185.3365, -21.0106) centre (185.3365, -17.8356) ccw projected
  line L11 (185.3365, -21.0106) -> (191.6865, -21.0106) projected
  arc A11 (191.6865, -21.0106) -> (194.8615, -17.8356) centre (191.6865, -17.8356) ccw projected
  circle A12 centre (103.8899, 44.3888) radius 1.524 projected
  circle A13 centre (83.8239, 44.3888) radius 1.524 projected
  circle A14 centre (103.8899, -1.2407) radius 1.524 projected
  circle A15 centre (83.8239, -1.2407) radius 1.524 projected
  circle A16 centre (159.7699, 44.3888) radius 1.524 projected
  circle A17 centre (139.7039, 44.3888) radius 1.524 projected
  circle A18 centre (159.7699, -1.2407) radius 1.524 projected
  circle A19 centre (139.7039, -1.2407) radius 1.524 projected
  circle A20 centre (187.7099, 44.3888) radius 1.524 projected
  circle A21 centre (167.6439, 44.3888) radius 1.524 projected
  circle A22 centre (187.7099, -1.2407) radius 1.524 projected
  circle A23 centre (167.6439, -1.2407) radius 1.524 projected
  circle A24 centre (111.7639, -1.2407) radius 1.524 projected
  circle A25 centre (131.8299, -1.2407) radius 1.524 projected
  circle A26 centre (111.7639, 44.3888) radius 1.524 projected
  circle A27 centre (131.8299, 44.3888) radius 1.524 projected
  circle A28 centre (55.8839, 44.3888) radius 1.524 projected
  circle A29 centre (75.9499, 44.3888) radius 1.524 projected
  circle A30 centre (55.8839, -1.2407) radius 1.524 projected
  circle A31 centre (75.9499, -1.2407) radius 1.524 projected
  line L12 (185.3365, -5.1356) -> (58.2572, -5.1356)
  line L13 (58.2572, -5.1356) -> (58.2572, -17.8356)
  line L14 (58.2572, -17.8356) -> (51.9072, -17.8356)
  line L15 (51.9072, -17.8356) -> (51.9072, 60.9837)
  line L16 (51.9072, 60.9837) -> (58.2572, 60.9837)
  line L17 (58.2572, 60.9837) -> (58.2572, 48.2837)
  line L18 (58.2572, 48.2837) -> (185.3365, 48.2837)
  line L19 (185.3365, 48.2837) -> (185.3365, 60.9837)
  line L20 (185.3365, 60.9837) -> (191.6865, 60.9837)
  line L21 (191.6865, 60.9837) -> (191.6865, -17.8356)
  line L22 (191.6865, -17.8356) -> (185.3365, -17.8356)
  line L23 (185.3365, -17.8356) -> (185.3365, -5.1356)
  line L24 (51.9072, -5.1356) -> (191.6865, -5.1356) projected
  line L25 (185.3365, -5.1356) -> (191.6865, -5.1356)
  line L26 (191.6865, -5.1356) -> (51.9072, -5.1356)
  line L27 (191.6865, 48.2837) -> (51.9072, 48.2837) projected
  line L28 (51.9072, -5.1356) -> (51.9072, 48.2837)
  line L29 (51.9072, 48.2837) -> (191.6865, 48.2837)
  point P0 (0, 0)
  dimension "d381" = 3.175
  constraints: 32 end point, 2 collinear, 1 perpendicular, 11 other
  measures "d381" distance between parallel lines of L9 L12
extrude "Extrusion10" add sketch "Sketch13" along normal blind 3.175 contours L21 L27 L19 A0 | A0 L20 L21 | A0 L19 L20 | L21 A3 L23 L24 | L27 L15 A1 L17 | L21 L22 A3 | A1 L16 L17 | A3 L22 L23 | L13 A2 L15 L24 | A1 L15 L16 | L13 L14 A2 | A2 L14 L15 | A11 L11 A10 L10 L9 L8 A9 L7 A8 L6 A7 L5 A6 L4 L3 L2 A5 L1 A4 L0
body "Solid1"
